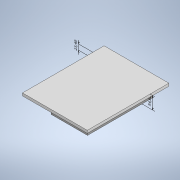
# Autodesk Inventor part: LCDScreen
Saved by Autodesk Inventor 2020 (Build 240168000, 168)
## iProperties
Created: 2019-07-11
Part Number: LCDScreen
Material: Generic
Document SubType Name: Modeling
Designer: El-KhouryJonathan
Density: 1 g/cm^3
Appearance: Default
Author: El-KhouryJonathan
Autodesk Inventor part; units mm, degrees
ref_plane "YZ Plane" through (0, 0, 0) normal (1, 0, 0) x (0, 1, 0)
ref_plane "XZ Plane" through (0, 0, 0) normal (0, 1, 0) x (-1, 0, 0)
ref_plane "XY Plane" through (0, 0, 0) normal (0, 0, 1) x (1, 0, 0)
sketch "Sketch1" plane through (0, 0, 0) normal (0, 1, 0) x (-1, 0, 0)
  point P0 (0, 0)
sketch "Sketch2" plane through (0, 0, 0) normal (0, 1, 0) x (-1, 0, 0)
  line L0 (-140.5, 177) -> (140.5, 177)
  line L1 (140.5, 177) -> (140.5, -177)
  line L2 (140.5, -177) -> (-140.5, -177)
  line L3 (-140.5, -177) -> (-140.5, 177)
  line L4 (-140.5, 177) -> (140.5, -177) construction
  line L5 (140.5, 177) -> (-140.5, -177) construction
  point P0 (0, 0)
  dimension "d0" = 354
  dimension "d1" = 281
  constraints: 12 end point, 2 midpoint, 2 parallel, 1 horizontal, 1 perpendicular
  measures "d0" distance of L0.end L1.end
  measures "d1" distance of L0.start L0.end
extrude "Extrusion1" add sketch "Sketch2" along normal blind 11.4
sketch "Sketch3" plane through (0, 0, 0) normal (0, -1, 0) x (1, 0, 0)
  line L0 (-124, -160.5) -> (125.8, -160.5)
  line L1 (125.8, -160.5) -> (125.8, 160.5)
  line L2 (125.8, 160.5) -> (-124, 160.5)
  line L3 (-124, 160.5) -> (-124, -160.5)
  line L4 (-123, -158.8) -> (123, 158.8) construction
  line L5 (123, -158.8) -> (-123, 158.8) construction
  circle A0 centre (-115.5, -152) radius 2
  circle A1 centre (117.3, -152) radius 2
  circle A2 centre (117.3, 152) radius 2
  circle A3 centre (-115.5, 152) radius 2
  line L6 (-140.5, -177) -> (-140.5, 177) projected
  line L7 (-140.5, 177) -> (140.5, 177) projected
  line L8 (140.5, -177) -> (-140.5, -177) projected
  line L9 (140.5, 177) -> (140.5, -177) projected
  circle A4 centre (-115.5, 0) radius 2
  circle A5 centre (117.3, 0) radius 2
  circle A6 centre (0, 152) radius 2
  circle A7 centre (0, -152) radius 2
  point P0 (0, 0)
  dimension "d189" = 4
  dimension "d190" = 8.5
  dimension "d191" = 8.5
  dimension "d192" = 8.5
  dimension "d193" = 8.5
  dimension "d194" = 8.5
  dimension "d195" = 8.5
  dimension "d196" = 8.5
  dimension "d197" = 8.5
  dimension "d207" = 16.5
  dimension "d208" = 16.5
  dimension "d209" = 16.5
  dimension "d210" = 14.7
  dimension "d211" = 8.5
  dimension "d212" = 354
  dimension "d213" = 177
  dimension "d214" = 8.5
  dimension "d215" = 177
  dimension "d216" = 8.5
  dimension "d217" = 281
  dimension "d218" = 140.5
  dimension "d220" = 140.5
  dimension "d221" = 8.5
  constraints: 12 end point, 8 centre point, 7 equal radius, 2 midpoint, 2 parallel, 1 horizontal, 1 perpendicular
  measures "d189" diameter of A0
  measures "d190" distance from line of L3 A0.centre
  measures "d191" distance from line of L0 A0.centre
  measures "d192" distance from line of L1 A1.centre
  measures "d193" distance from line of L0 A1.centre
  measures "d194" distance from line of L1 A2.centre
  measures "d195" distance from line of L2 A2.centre
  measures "d196" distance from line of L2 A3.centre
  measures "d197" distance from line of L3 A3.centre
  measures "d207" distance between parallel lines of L6 L3
  measures "d208" distance between parallel lines of L7 L2
  measures "d209" distance between parallel lines of L8 L0
  measures "d210" distance between parallel lines of L9 L1
  measures "d211" distance from line of L3 A4.centre
  measures "d212" distance of L6.start L6.end
  measures "d213" distance from line of L7 A4.centre
  measures "d214" distance from line of L1 A5.centre
  measures "d215" distance from line of L7 A5.centre
  measures "d216" distance from line of L2 A6.centre
  measures "d217" distance of L6.end L7.end
  measures "d218" distance from line of L9 A6.centre
  measures "d220" distance from line of L9 A7.centre
  measures "d221" distance from line of L0 A7.centre
extrude "Extrusion2" add sketch "Sketch3" along normal blind 12 contours L3 L2 L1 L0
sketch "Sketch7" plane through (0, -12, 0) normal (0, -1, 0) x (1, 0, 0)
  line L0 (-52.5, 141) -> (105.5, 141)
  line L1 (105.5, 141) -> (105.5, -141)
  line L2 (105.5, -141) -> (-52.5, -141)
  line L3 (-52.5, -141) -> (-52.5, 141)
  line L4 (-52.5, 141) -> (105.5, -141) construction
  line L5 (105.5, 141) -> (-52.5, -141) construction
  line L6 (125.8, -160.5) -> (125.8, 160.5) projected
  line L7 (-124, -160.5) -> (125.8, -160.5) projected
  line L8 (-140.5, 177) -> (140.5, 177) projected
  line L9 (140.5, -177) -> (-140.5, -177) projected
  line L10 (140.5, 177) -> (140.5, -177) projected
  point P0 (0, 0)
  dimension "d62" = 158
  dimension "d204" = 36
  dimension "d205" = 36
  dimension "d206" = 35
  constraints: 12 end point, 2 parallel, 1 horizontal, 1 perpendicular
  measures "d62" distance of L0.start L0.end
  measures "d204" distance between parallel lines of L8 L0
  measures "d205" distance between parallel lines of L9 L2
  measures "d206" distance between parallel lines of L10 L1
extrude "Extrusion3" add sketch "Sketch7" along normal blind 31.2
sketch "Sketch8" plane through (0, -43.2, 0) normal (0, -1, 0) x (1, 0, 0)
  line L0 (99.2, 131) -> (81.2, 131)
  line L1 (81.2, 131) -> (81.2, 15)
  line L2 (81.2, 15) -> (99.2, 15)
  line L3 (99.2, 15) -> (99.2, 131)
  line L4 (99.2, 131) -> (81.2, 15) construction
  line L5 (81.2, 131) -> (99.2, 15) construction
  line L6 (105.5, -141) -> (105.5, 141) projected
  line L7 (105.5, 141) -> (-52.5, 141) projected
  point P0 (0, 0)
  point P1 (90.2, 73)
  dimension "d67" = 116
  dimension "d68" = 18
  dimension "d69" = 6.3
  dimension "d70" = 10
  constraints: 12 end point, 2 midpoint, 2 parallel, 1 horizontal, 1 perpendicular
  measures "d67" distance of L0.end L1.end
  measures "d68" distance of L1.end L2.end
  measures "d69" distance between parallel lines of L6 L3
  measures "d70" distance between parallel lines of L7 L0
extrude "Extrusion4" add sketch "Sketch8" along normal blind 1
sketch "Sketch9" plane through (0, -43.2, 0) normal (0, -1, 0) x (1, 0, 0)
  line L0 (100, -71.4) -> (42.15, -71.4)
  line L1 (42.15, -71.4) -> (42.15, -129.25)
  line L2 (42.15, -129.25) -> (100, -129.25)
  line L3 (100, -129.25) -> (100, -71.4)
  line L4 (100, -71.4) -> (42.15, -129.25) construction
  line L5 (42.15, -71.4) -> (100, -129.25) construction
  line L6 (105.5, -141) -> (105.5, 141) projected
  line L7 (-52.5, -141) -> (105.5, -141) projected
  point P0 (0, 0)
  point P1 (71.075, -100.325)
  dimension "d73" = 5.5
  dimension "d74" = 57.85
  dimension "d75" = 11.75
  dimension "d76" = 57.85
  constraints: 12 end point, 2 midpoint, 2 parallel, 1 horizontal, 1 perpendicular
  measures "d73" distance between parallel lines of L3 L6
  measures "d74" distance of L2.end L0.start
  measures "d75" distance between parallel lines of L7 L2
  measures "d76" distance of L0.start L0.end
extrude "Extrusion5" add sketch "Sketch9" along normal blind 1
sketch "Sketch10" plane through (0, -43.2, 0) normal (0, -1, 0) x (1, 0, 0)
  line L0 (105.5, 141) -> (-52.5, 141) projected
  line L1 (-52.5, 141) -> (-52.5, -141) projected
  line L2 (-52.5, -141) -> (105.5, -141) projected
  point P0 (0, 0)
  point P1 (-45.5, 120.2)
  point P2 (-45.5, -119.9)
  dimension "d86" = 20.8
  dimension "d87" = 7
  dimension "d90" = 240.1
  dimension "d95" = 21.1
  constraints: 1 vertical, 1 other
  measures "d86" distance from line of L0 point (-45.5, 120.2)
  measures "d87" distance from line of L1 point (-45.5, 120.2)
  measures "d90" distance of point (-45.5, 120.2) point (-45.5, -119.9)
  measures "d95" distance from line of L2 point (-45.5, -119.9)
hole "Hole4" at (-45.5, -43.2, 120.2) at (-45.5, -43.2, -119.9) direction (0, 1, 0) diameter 7 depth 8 tip angle 118
sketch "Sketch11" plane through (0, -43.2, 0) normal (0, -1, 0) x (1, 0, 0)
  line L0 (105.5, 141) -> (-52.5, 141) projected
  line L1 (-52.5, 141) -> (-52.5, -141) projected
  line L2 (125.8, 160.5) -> (-124, 160.5) projected
  point P0 (0, 0)
  point P1 (-45.5, 0)
  dimension "d103" = 141
  dimension "d104" = 7
  dimension "d185" = 160.5
  measures "d103" distance from line of point (-45.5, 0) L0
  measures "d104" distance from line of L1 point (-45.5, 0)
  measures "d185" distance from line of point (-45.5, 0) L2
hole "Hole5" at (-45.5, -43.2, 0) direction (0, 1, 0) diameter 7 depth 8 tip angle 118
sketch "Sketch12" plane through (0, -43.2, 0) normal (0, -1, 0) x (1, 0, 0)
  line L0 (105.5, 141) -> (-52.5, 141) projected
  line L1 (-52.5, 141) -> (-52.5, -141) projected
  point P0 (0, 0)
  point P1 (-18.7, 37.65)
  point P2 (-18.7, -36.85)
  point P3 (55.8, 37.65)
  point P4 (55.8, -36.85)
  dimension "d112" = 103.35
  dimension "d113" = 33.8
  dimension "d116" = 74.5
  dimension "d119" = 74.5
  constraints: 1 horizontal, 1 vertical, 3 other
  measures "d112" distance from line of L0 point (-18.7, 37.65)
  measures "d113" distance from line of L1 point (-18.7, 37.65)
  measures "d116" distance of point (-18.7, 37.65) point (-18.7, -36.85)
  measures "d119" distance of point (-18.7, 37.65) point (55.8, 37.65)
hole "Hole6" at (-18.7, -43.2, 37.65) at (55.8, -43.2, 37.65) at (55.8, -43.2, -36.85) at (-18.7, -43.2, -36.85) direction (0, 1, 0) diameter 7 depth 8 tip angle 118
sketch "Sketch13" plane through (-52.5, -12, -141) normal (-1, 0, 0) x (0, 0, 1)
  line L0 (223, -24.2) -> (195.5, -24.2)
  line L1 (195.5, -24.2) -> (195.5, -2.2)
  line L2 (195.5, -2.2) -> (223, -2.2)
  line L3 (223, -2.2) -> (223, -24.2)
  line L4 (223, -24.2) -> (195.5, -2.2) construction
  line L5 (195.5, -24.2) -> (223, -2.2) construction
  line L6 (282, 0) -> (282, -31.2) projected
  line L7 (282, -31.2) -> (0, -31.2) projected
  point P0 (141, 12)
  point P1 (209.25, -13.2)
  dimension "d122" = 59
  dimension "d123" = 27.5
  dimension "d124" = 22
  dimension "d133" = 7
  constraints: 12 end point, 2 midpoint, 2 parallel, 1 horizontal, 1 perpendicular
  measures "d122" distance between parallel lines of L6 L3
  measures "d123" distance of L0.start L0.end
  measures "d124" distance of L0.end L1.end
  measures "d133" distance between parallel lines of L7 L0
extrude "Extrusion6" cut sketch "Sketch13" against normal blind 10
sketch "Sketch14" plane through (-52.5, -12, -141) normal (-1, 0, 0) x (0, 0, 1)
  line L0 (142, -11.8) -> (125, -11.8)
  line L1 (125, -11.8) -> (125, -5.6)
  line L2 (125, -5.6) -> (142, -5.6)
  line L3 (142, -5.6) -> (142, -11.8)
  line L4 (142, -11.8) -> (125, -5.6) construction
  line L5 (125, -11.8) -> (142, -5.6) construction
  line L6 (195.5, -24.2) -> (195.5, -2.2) projected
  line L7 (282, -31.2) -> (0, -31.2) projected
  line L8 (223, -24.2) -> (195.5, -24.2) projected
  line L9 (301.5, 0) -> (-19.5, 0) projected
  line L10 (195.5, -2.2) -> (223, -2.2) projected
  line L11 (282, 0) -> (282, -31.2) projected
  point P0 (141, 12)
  point P1 (133.5, -8.7)
  dimension "d128" = 6.2
  dimension "d129" = 17
  dimension "d130" = 19.4
  dimension "d222" = 140
  constraints: 12 end point, 2 midpoint, 2 parallel, 1 horizontal, 1 perpendicular
  measures "d128" distance of L2.end L0.start
  measures "d129" distance of L0.start L0.end
  measures "d130" distance between parallel lines of L7 L0
  measures "d222" distance between parallel lines of L11 L3
extrude "Extrusion7" cut sketch "Sketch14" against normal blind 1.5
sketch "Sketch15" plane through (-52.5, -12, -141) normal (-1, 0, 0) x (0, 0, 1)
  line L0 (118, -11.8) -> (103, -11.8)
  line L1 (103, -11.8) -> (103, -5.6)
  line L2 (103, -5.6) -> (118, -5.6)
  line L3 (118, -5.6) -> (118, -11.8)
  line L4 (118, -11.8) -> (103, -5.6) construction
  line L5 (103, -11.8) -> (118, -5.6) construction
  line L6 (125, -11.8) -> (125, -5.6) projected
  line L7 (282, -31.2) -> (0, -31.2) projected
  point P0 (141, 12)
  point P1 (110.5, -8.7)
  dimension "d136" = 7
  dimension "d137" = 6.2
  dimension "d138" = 15
  dimension "d141" = 19.4
  constraints: 12 end point, 2 midpoint, 2 parallel, 1 horizontal, 1 perpendicular
  measures "d136" distance between parallel lines of L3 L6
  measures "d137" distance of L0.end L1.end
  measures "d138" distance of L0.start L0.end
  measures "d141" distance between parallel lines of L7 L0
extrude "Extrusion8" cut sketch "Sketch15" against normal blind 1.5
sketch "Sketch16" plane through (-52.5, -12, -141) normal (-1, 0, 0) x (0, 0, 1)
  circle A0 centre (92.5, -12.2) radius 2.5
  line L0 (103, -11.8) -> (103, -5.6) projected
  line L1 (282, -31.2) -> (0, -31.2) projected
  circle A1 centre (68, -12.2) radius 2.5
  line L2 (88.375, -16.2) -> (72.125, -16.2)
  line L3 (72.125, -16.2) -> (72.125, -8.2)
  line L4 (72.125, -8.2) -> (88.375, -8.2)
  line L5 (88.375, -8.2) -> (88.375, -16.2)
  line L6 (88.375, -16.2) -> (72.125, -8.2) construction
  line L7 (72.125, -16.2) -> (88.375, -8.2) construction
  point P0 (141, 12)
  point P1 (80.25, -12.2)
  dimension "d142" = 10.5
  dimension "d144" = 5
  dimension "d147" = 24.5
  dimension "d223" = 19
  dimension "d224" = 12.25
  dimension "d225" = 19
  dimension "d226" = 16.25
  dimension "d227" = 8
  constraints: 12 end point, 2 centre point, 2 horizontal, 2 midpoint, 2 parallel, 1 perpendicular, 2 other
  measures "d142" distance from line of A0.centre L0
  measures "d144" diameter of A0
  measures "d147" distance of A0.centre A1.centre
  measures "d223" distance from line of L1 A0.centre
  measures "d224" distance of A0.centre point (80.25, -12.2)
  measures "d225" distance from line of L1 point (80.25, -12.2)
  measures "d226" distance of L2.start L2.end
  measures "d227" distance of L2.end L3.end
extrude "Extrusion9" add sketch "Sketch16" along normal blind 5
sketch "Sketch20" plane through (0, -12, 0) normal (0, -1, 0) x (1, 0, 0)
  circle A0 centre (-59, 120) radius 2
  circle A1 centre (-59, 0) radius 2
  circle A2 centre (-59, -120) radius 2
  line L0 (-52.5, -141) -> (-52.5, 141) projected
  circle A3 centre (-115.5, 152) radius 2 projected
  point P0 (0, 0)
  dimension "d228" = 21
  dimension "d229" = 6.5
  dimension "d230" = 6.5
  dimension "d231" = 6.5
  dimension "d232" = 21
  dimension "d233" = 240
  dimension "d234" = 120
  constraints: 3 centre point, 3 equal radius
  measures "d228" vertical distance of L0.end A0.centre
  measures "d229" distance from line of L0 A0.centre
  measures "d230" distance from line of L0 A1.centre
  measures "d231" distance from line of L0 A2.centre
  measures "d232" vertical distance of L0.start A2.centre
  measures "d233" distance of A2.centre A0.centre
  measures "d234" distance of A0.centre A1.centre
extrude "Extrusion11" cut sketch "Sketch20" against normal blind 10 contours A0 | A1 | A2
equation "\"d191\" = d190"
equation "\"d192\" = d190"
equation "\"d193\" = d190"
equation "\"d194\" = d190"
equation "\"d195\" = d190"
equation "\"d196\" = d190"
equation "\"d197\" = d190"
equation "\"d209\" = d208"
equation "\"d211\" = d190"
equation "\"d213\" = 0.5 * d212"
equation "\"d214\" = d190"
equation "\"d215\" = d213"
equation "\"d216\" = d190"
equation "\"d218\" = 0.5 * d217"
equation "\"d220\" = d218"
equation "\"d221\" = d190"
equation "\"d205\" = d204"
equation "\"d224\" = 0.5 * d147"
equation "\"d225\" = d223"
equation "\"d230\" = d229"
equation "\"d231\" = d229"
equation "\"d232\" = d228"
equation "\"d234\" = 0.5 * d233"
body "Solid1"
